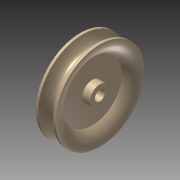
# Autodesk Inventor part: pulley wheel
Saved by Autodesk Inventor 2014 (Build 180170000, 170)
## iProperties
Created: 2013-10-13
Part Number: pulley wheel
Material: Polyethylene, Low Density
Document SubType Name: Modeling
Designer: david
Density: 0.894 g/cm^3
Appearance: Smooth - Off-White
Author: david
Autodesk Inventor part; units mm, degrees
ref_plane "YZ Plane" through (0, 0, 0) normal (1, 0, 0) x (0, 1, 0)
ref_plane "XZ Plane" through (0, 0, 0) normal (0, 1, 0) x (-1, 0, 0)
ref_plane "XY Plane" through (0, 0, 0) normal (0, 0, 1) x (1, 0, 0)
sketch "Sketch1" plane through (0, 0, 0) normal (0, 1, 0) x (-1, 0, 0)
  line L0 (0, 0) -> (12.7, 0)
  line L1 (12.7, 0) -> (12.7, 6.35)
  line L2 (0, 6.35) -> (0, 0)
  spline S0 degree 2 poles (1.5875, 28.575) (6.35, 15.892) (11.1125, 28.575) knots 0 0 0 1 1 1
  line L3 (12.7, 6.35) -> (12.7, 0)
  line L4 (0, 6.35) -> (0, 0)
  line L5 (12.7, 28.575) -> (11.1125, 28.575)
  line L6 (1.5875, 28.575) -> (0, 28.575)
  arc A0 (8.0957, 19.05) -> (12.7, 28.575) centre (0.5456, 28.575) ccw
  arc A1 (0, 28.575) -> (4.9207, 19.05) centre (12.152, 28.8193) ccw
  line L7 (4.9207, 19.05) -> (4.9207, 6.35)
  line L8 (8.0957, 19.05) -> (8.0957, 6.35)
  line L9 (0, 6.35) -> (4.9207, 6.35)
  line L10 (8.0957, 6.35) -> (12.7, 6.35)
  point P0 (6.35, 22.2335)
  dimension "d0" = 12.7
  dimension "d1" = 28.575
  dimension "d7" = 1.5875
  dimension "d8" = 1.5875
  dimension "d12" = 3.175
  dimension "d14" = 6.35
  dimension "d15" = 6.35
  constraints: 22 end point, 7 perpendicular, 4 point on circle, 3 parallel, 2 centre point, 2 horizontal, 1 equal radius, 1 tangent, 5 other
  measures "d0" distance of L0.start L0.end
  measures "d1" distance of L6.end L0.start
  measures "d7" distance from line of L2 L6.start
  measures "d8" distance from line of L1 L5.end
  measures "d12" distance of L8.start L7.start
  measures "d14" distance of L0.end L1.end
  measures "d15" distance of L2.start L0.start
revolve "Revolution1" add sketch "Sketch1" angle 360 about axis through (0, 0, 0) along (-1, 0, 0)
sketch "Sketch2" plane through (0, 0, 0) normal (1, 0, 0) x (0, 0, -1)
  circle A0 centre (0, 0) radius 6.35 projected
  constraints: 1 coincident
hole "Hole1" at (0, 0, 0) direction (-1, 0, 0) diameter 6.35 end through all
body "Solid1"
